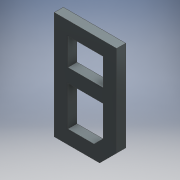
# Autodesk Inventor part: chassi_back_template
Saved by Autodesk Inventor 2016 (Build 200138000, 138)
## iProperties
Created: 2017-01-03
Part Number: chassi_back_template
Material: Generic
Document SubType Name: Modeling
Designer: hesaon
Density: 1 g/cm^3
Appearance: Default
Author: hesaon
Autodesk Inventor part; units mm, degrees
ref_plane "YZ Plane" through (0, 0, 0) normal (1, 0, 0) x (0, 1, 0)
ref_plane "XZ Plane" through (0, 0, 0) normal (0, 1, 0) x (-1, 0, 0)
ref_plane "XY Plane" through (0, 0, 0) normal (0, 0, 1) x (1, 0, 0)
sketch "Sketch1" plane through (0, 0, 0) normal (0, 1, 0) x (-1, 0, 0)
  line L0 (0, 142.5) -> (0, 0)
  line L1 (0, 142.5) -> (-82.5, 142.5)
  line L2 (0, 0) -> (-60, 0)
  line L3 (-60, 0) -> (-82.5, 22.5)
  line L4 (-82.5, 142.5) -> (-82.5, 22.5)
  line L5 (-18, 18) -> (-52.5442, 18)
  line L6 (-64.5, 124.5) -> (-18, 124.5)
  line L7 (-18, 88.5) -> (-64.5, 88.5)
  line L8 (-18, 70.5) -> (-64.5, 70.5)
  line L9 (-18, 124.5) -> (-18, 88.5)
  line L10 (-18, 70.5) -> (-18, 18)
  line L11 (-64.5, 29.9558) -> (-64.5, 70.5)
  line L12 (-64.5, 88.5) -> (-64.5, 124.5)
  line L13 (-52.5442, 18) -> (-64.5, 29.9558)
  dimension "d1" = 142.5
  dimension "d3" = 82.5
  dimension "d4" = 60
  dimension "d5" = 135
  dimension "d6" = 120
  dimension "d8" = 18
  dimension "d9" = 18
  dimension "d15" = 88.5
  dimension "d16" = 18
  dimension "d17" = 18
  dimension "d18" = 18
  dimension "d19" = 18
  dimension "d20" = 18
  dimension "d21" = 18
  constraints: 28 end point, 6 perpendicular, 3 vertical, 2 horizontal, 2 parallel, 1 coincident
  measures "d1" distance of L0.end L0.start
  measures "d3" distance of L0.start L1.end
  measures "d4" distance of L0.end L2.end
  measures "d5" angle of L2 L3
  measures "d6" distance of L3.end L1.end
  measures "d8" distance between parallel lines of L1 L6
  measures "d9" distance between parallel lines of L2 L5
  measures "d15" distance between parallel lines of L2 L7
  measures "d16" distance between parallel lines of L8 L7
  measures "d17" distance of L8.end L7.end
  measures "d18" distance from line of L0 L6.end
  measures "d19" distance between parallel lines of L0 L10
  measures "d20" distance between parallel lines of L4 L12
  measures "d21" distance between parallel lines of L3 L13
extrude "Extrusion2" add sketch "Sketch1" along normal blind 12
body "Solid2"
